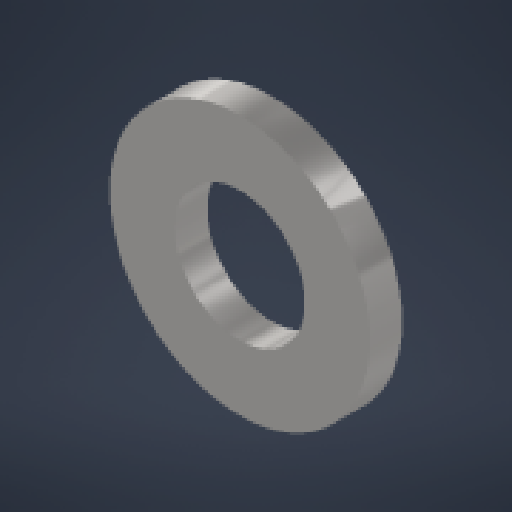
# Autodesk Inventor part: E-GPWSSS12-4-1
Saved by Autodesk Inventor 2024.3 (Build 283343000, 343)
## iProperties
Part Number: E-GPWSSS12-4-1
Material: ステンレス鋼 AISI 304
Catalog Web Link: https://www.hirosugi-net.co.jp/shop/g/g58928/
Description: ReadyMade
Document SubType Name: Modeling
Designer: ASUS
Mass: 0.71145 g
Surface Area: 3.00273 cm^2
Volume: 0.198486 cm^3
Density: 3.58439 g/cm^3
Appearance: 半つや出し
Author: Masato Kubotera
Autodesk Inventor part; units mm, degrees
ref_plane "YZ Plane" through (0, 0, 0) normal (1, 0, 0) x (0, 1, 0)
ref_plane "XZ Plane" through (0, 0, 0) normal (0, 1, 0) x (-1, 0, 0)
ref_plane "XY Plane" through (0, 0, 0) normal (0, 0, 1) x (1, 0, 0)
sketch "スケッチ1" plane through (0, 0, 0) normal (0, 0, 1) x (1, 0, 0)
  circle A0 centre (0, 0) radius 2
  circle A1 centre (0, 0) radius 4
  dimension "d0" = 4
  dimension "d1" = 8
  constraints: 2 centre point, 2 coincident
  measures "d0" diameter of A0
  measures "d1" diameter of A1
extrude "押し出し1" add sketch "スケッチ1" along normal blind 1
